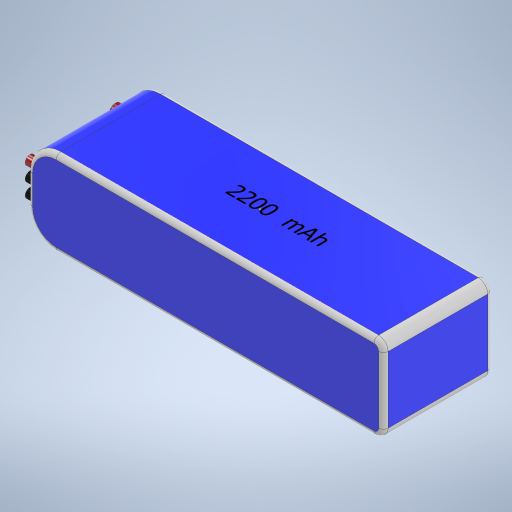
# Autodesk Inventor part: bateria
Saved by Autodesk Inventor 2023 (Build 270158000, 158)
## iProperties
Created: 2023-08-10
Part Number: bateria
Material: Genérico
Document SubType Name: Modeling
Designer: azeve
Density: 1 g/cm^3
Appearance: Padrão
Author: azeve
Autodesk Inventor part; units mm, degrees
ref_plane "YZ Plane" through (0, 0, 0) normal (1, 0, 0) x (0, 1, 0)
ref_plane "XZ Plane" through (0, 0, 0) normal (0, 1, 0) x (-1, 0, 0)
sketch "Esboço1" plane through (0, 0, 0) normal (0, 1, 0) x (-1, 0, 0)
  line L0 (-37.5, 11.5) -> (37.5, 11.5)
  line L1 (37.5, 11.5) -> (37.5, -11.5)
  line L2 (37.5, -11.5) -> (-37.5, -11.5)
  line L3 (-37.5, -11.5) -> (-37.5, 11.5)
  line L4 (-37.5, 11.5) -> (37.5, -11.5) construction
  line L5 (37.5, 11.5) -> (-37.5, -11.5) construction
  point P0 (0, 0)
  dimension "d0" = 75
  dimension "d1" = 23
  constraints: 12 end point, 2 midpoint, 2 parallel, 1 horizontal, 1 perpendicular
  measures "d0" distance of L1.end L2.end
  measures "d1" distance of L0.end L1.end
extrude "Extrusão1" add sketch "Esboço1" along normal blind 18
fillet "Arredondamento1" radius 6 2 edges at (-37.5, 18, 0) (-37.5, 0, 0)
ref_plane "Plano de trabalho1" through (-37.5, 6, 11.5) normal (-1, 0, 0) x (0, 0, 1)
sketch "Esboço2" plane through (-37.5, 6, 11.5) normal (-1, 0, 0) x (0, 0, 1)
  line L0 (-23, -6) -> (-23, 12) projected
  line L1 (-23, 3) -> (-17.6681, 8.7956) construction
  line L2 (-19.3047, -1.0167) -> (-21.1754, 1.0167) construction
  line L3 (-23, -2.7956) -> (-23, 8.7956)
  line L4 (0, 0) -> (-23, 0) projected
  circle A0 centre (-20.24, 0) radius 1.3815
  line L5 (-23, 6) -> (0, 6) projected
  circle A1 centre (-20.24, 6) radius 1.3706
  circle A2 centre (-2.2088, 3) radius 1.0065
  circle A3 centre (-2.2088, 6) radius 1
  circle A4 centre (-2.2088, 0) radius 1
  point P0 (-11.5, -6)
  dimension "d6" = 2
  dimension "d7" = 2
  constraints: 7 point on line, 6 end point, 5 centre point, 2 midpoint, 2 point on circle, 1 collinear
  measures "d6" diameter of A3
  measures "d7" diameter of A4
extrude "Extrusão2" add sketch "Esboço2" along normal blind 1.75
fillet "Arredondamento2" radius 2 2 edges at (37.5, 18, 0) (37.5, 0, 0)
fillet "Arredondamento3" radius 1 16 edges at (36.9142, 17.4142, 11.5) (37.5, 9, 11.5) (36.9142, 0.5858, 11.5) (2, 0, 11.5) (-35.7426, 1.7574, 11.5) (-37.5, 9, 11.5) (-35.7426, 16.2426, 11.5) (2, 18, 11.5) (-35.7426, 1.7574, -11.5) (-37.5, 9, -11.5) (-35.7426, 16.2426, -11.5) (2, 18, -11.5) (36.9142, 17.4142, -11.5) (37.5, 9, -11.5) (36.9142, 0.5858, -11.5) (2, 0, -11.5)
sketch "Esboço3" plane through (0, 18, 0) normal (0, 1, 0) x (1, 0, 0)
  line L0 (-29.9595, -10.4813) -> (30.9762, -10.4813) construction
  line L1 (-6.9418, 2.4664) -> (12.8628, 2.4664) construction
  line L2 (12.8628, 2.4664) -> (12.8628, -1.4881) construction
  line L3 (12.8628, -1.4881) -> (-6.9418, -1.4881) construction
  line L4 (-6.9418, -1.4881) -> (-6.9418, 2.4664) construction
  point P0 (0, 0)
  constraints: 2 end point, 1 horizontal, 2 other
